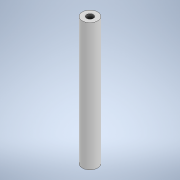
# Autodesk Inventor part: Connectors
Saved by Autodesk Inventor 2022 (Build 260153000, 153)
## iProperties
Created: 2023-03-10
Part Number: Connectors
Material: Generic
Document SubType Name: Modeling
Designer: zarek
Density: 1 g/cm^3
Appearance: Default
Author: zarek
Autodesk Inventor part; units mm, degrees
ref_plane "YZ Plane" through (0, 0, 0) normal (1, 0, 0) x (0, 1, 0)
ref_plane "XZ Plane" through (0, 0, 0) normal (0, 1, 0) x (-1, 0, 0)
ref_plane "XY Plane" through (0, 0, 0) normal (0, 0, 1) x (1, 0, 0)
sketch "Sketch1" plane through (0, 0, 0) normal (0, 1, 0) x (-1, 0, 0)
  circle A0 centre (0, 0) radius 3.5
  dimension "d0" = 7
  constraints: 1 centre point, 1 coincident
  measures "d0" diameter of A0
extrude "Extrusion1" add sketch "Sketch1" along normal blind 57.5
sketch "Sketch2" plane through (0, 57.5, 0) normal (0, 1, 0) x (1, 0, 0)
  circle A0 centre (0, 0) radius 0.9252
  constraints: 1 centre point, 1 coincident
hole "Hole1" at (0, 57.5, 0) direction (0, -1, 0) diameter 2.85 depth 19.05 tip angle 118 countersink diameter 3.048 countersink angle 82 thread size "M3.5x0.6" class "6H" standard "ANSI Metric M Profile"
sketch "Sketch3" plane through (0, 0, 0) normal (0, -1, 0) x (1, 0, 0)
  circle A0 centre (0, 0) radius 1.2742
  constraints: 1 centre point, 1 coincident
hole "Hole2" at (0, 0, 0) direction (0, 1, 0) diameter 2.85 depth 19.05 tip angle 118 countersink diameter 3.048 countersink angle 82 thread size "M3.5x0.6" class "6H" standard "ANSI Metric M Profile"
body "Solid1"
